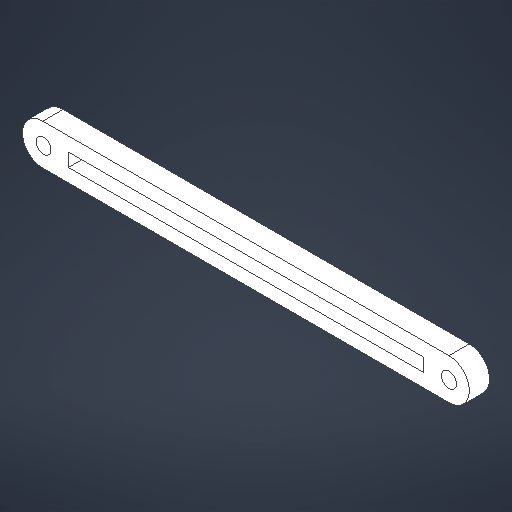
# Autodesk Inventor part: Bracket
Saved by Autodesk Inventor 2026.1 (Build 301233020, 233B)
## iProperties
Created: 2025-11-25
Part Number: Bracket
Material: Generic
Document SubType Name: Modeling
Designer: sarab
Density: 1 g/cm^3
Appearance: Default
Author: sarab
Autodesk Inventor part; units mm, degrees
ref_plane "YZ Plane" through (0, 0, 0) normal (1, 0, 0) x (0, 1, 0)
ref_plane "XZ Plane" through (0, 0, 0) normal (0, 1, 0) x (-1, 0, 0)
ref_plane "XY Plane" through (0, 0, 0) normal (0, 0, 1) x (1, 0, 0)
sketch "Sketch1" plane through (0, 0, 0) normal (0, 0, 1) x (1, 0, 0)
  line L0 (-111.7609, 28.9288) -> (-11.7609, 28.9288)
  line L1 (-11.7609, 28.9288) -> (-11.7609, 18.9288)
  line L2 (-11.7609, 18.9288) -> (-111.7609, 18.9288)
  line L3 (-111.7609, 18.9288) -> (-111.7609, 28.9288)
  arc A0 (-111.7609, 28.9288) -> (-111.7609, 18.9288) centre (-111.7609, 23.9288) ccw
  arc A1 (-11.7609, 18.9288) -> (-11.7609, 28.9288) centre (-11.7609, 23.9288) ccw
  point P0 (0, 0)
  point P1 (-105.9495, 22.4367)
  constraints: 8 end point, 4 point on circle, 2 centre point, 2 midpoint, 2 parallel, 2 point on line, 2 tangent, 1 horizontal, 1 perpendicular
extrude "Extrusion1" add sketch "Sketch1" along normal blind 5
sketch "Sketch2" plane through (0, 0, 5) normal (0, 0, 1) x (1, 0, 0)
  circle A0 centre (-11.7633, 23.7843) radius 1.841
  circle A1 centre (-111.5799, 23.7843) radius 1.841
  point P0 (0, 0)
  constraints: 2 centre point
extrude "Extrusion2" cut sketch "Sketch2" against normal blind 5
sketch "Sketch3" plane through (0, 0, 5) normal (0, 0, 1) x (1, 0, 0)
  line L0 (-105.444, 25.5006) -> (-17.9751, 25.5006)
  line L1 (-17.9751, 25.5006) -> (-17.9751, 22.2171)
  line L2 (-17.9751, 22.2171) -> (-105.444, 22.2171)
  line L3 (-105.444, 22.2171) -> (-105.444, 25.5006)
  point P0 (0, 0)
  constraints: 8 end point, 3 perpendicular, 1 horizontal
extrude "Extrusion3" cut sketch "Sketch3" against normal blind 10
body "Solid1"
